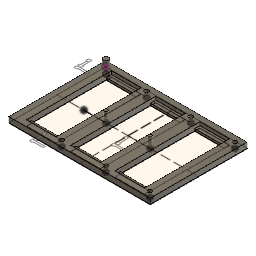
3Slideholder v1 (Autodesk Fusion 360 design; units mm, degrees)
Autodesk Fusion 360 part; units mm, degrees
note: some values were not read from the file. Set by a fixed rule: which sketch regions a step uses.
sketch "Sketch1" plane through (0, 0, 0) normal (0, 1, 0) x (1, 0, 0)
  line L0 (0, 0) -> (127.5, 0)
  line L1 (127.5, 0) -> (127.5, -87.5)
  line L2 (127.5, -87.5) -> (0, -87.5)
  line L3 (0, -87.5) -> (0, 0)
  line L4 (0, -43.75) -> (127.5, -43.75) construction
  line L5 (63.75, 0) -> (63.75, -87.5) construction
  line L6 (63.75, -43.75) -> (77.05, -43.75) construction
  line L7 (63.75, -43.75) -> (63.75, -5.45) construction
  line L8 (63.75, -5.45) -> (77.05, -5.45) construction
  line L9 (77.05, -5.45) -> (50.45, -5.45)
  line L10 (50.45, -5.45) -> (50.45, -82.05)
  line L11 (50.45, -82.05) -> (77.05, -82.05)
  line L12 (77.05, -82.05) -> (77.05, -5.45)
  line L13 (50.45, -43.75) -> (37.25, -43.75)
  line L14 (37.25, -43.75) -> (37.25, -5.45)
  line L15 (37.25, -5.45) -> (10.65, -5.45)
  line L16 (10.65, -5.45) -> (10.65, -82.05)
  line L17 (10.65, -82.05) -> (37.25, -82.05)
  line L18 (37.25, -82.05) -> (37.25, -5.45)
  line L19 (77.05, -43.75) -> (90.25, -43.75)
  line L20 (90.25, -43.75) -> (90.25, -5.45)
  line L21 (90.25, -5.45) -> (116.85, -5.45)
  line L22 (116.85, -5.45) -> (116.85, -82.05)
  line L23 (116.85, -82.05) -> (90.25, -82.05)
  line L24 (90.25, -82.05) -> (90.25, -5.45)
  line L25 (37.25, -43.75) -> (23.95, -43.75)
  line L26 (37.25, -5.45) -> (37.25, -10.2)
  line L27 (37.25, -10.2) -> (10.65, -10.2)
  line L28 (10.65, -10.2) -> (10.65, -5.45)
  line L29 (10.65, -5.45) -> (37.25, -5.45)
  line L30 (37.25, -5.45) -> (37.25, -10.2)
  line L31 (50.45, -5.45) -> (50.45, -10.2)
  line L32 (50.45, -10.2) -> (77.05, -10.2)
  line L33 (77.05, -10.2) -> (77.05, -5.45)
  line L34 (77.05, -5.45) -> (50.45, -5.45)
  line L35 (50.45, -5.45) -> (50.45, -10.2)
  line L36 (90.25, -5.45) -> (90.25, -10.2)
  line L37 (90.25, -10.2) -> (116.85, -10.2)
  line L38 (116.85, -10.2) -> (116.85, -5.45)
  line L39 (116.85, -5.45) -> (90.25, -5.45)
  line L40 (90.25, -5.45) -> (90.25, -10.2)
  line L41 (10.65, -82.05) -> (37.25, -82.05)
  line L42 (37.25, -82.05) -> (37.25, -77.3)
  line L43 (37.25, -77.3) -> (10.65, -77.3)
  line L44 (10.65, -77.3) -> (10.65, -82.05)
  line L45 (50.45, -82.05) -> (77.05, -82.05)
  line L46 (77.05, -82.05) -> (77.05, -77.3)
  line L47 (77.05, -77.3) -> (50.45, -77.3)
  line L48 (50.45, -77.3) -> (50.45, -82.05)
  line L49 (116.85, -82.05) -> (90.25, -82.05)
  line L50 (90.25, -82.05) -> (90.25, -77.3)
  line L51 (90.25, -77.3) -> (116.85, -77.3)
  line L52 (116.85, -77.3) -> (116.85, -82.05)
  line L53 (77.05, -43.75) -> (83.65, -43.75)
  circle A0 centre (83.65, -43.75) radius 1.5
  line L54 (37.25, -43.75) -> (43.85, -43.75)
  circle A1 centre (43.85, -43.75) radius 1.5
  line L55 (10.65, -5.45) -> (5.65, -5.45)
  circle A2 centre (5.65, -5.45) radius 2.5
  line L56 (37.25, -5.45) -> (42.25, -5.45)
  circle A3 centre (42.25, -5.45) radius 1.875
  line L57 (77.05, -5.45) -> (82.05, -5.45)
  circle A4 centre (82.05, -5.45) radius 1.875
  line L58 (116.85, -5.45) -> (121.85, -5.45)
  circle A5 centre (121.85, -5.45) radius 1.875
  line L59 (116.85, -82.05) -> (121.85, -82.05)
  circle A6 centre (121.85, -82.05) radius 1.875
  line L60 (77.05, -82.05) -> (82.05, -82.05)
  circle A7 centre (82.05, -82.05) radius 1.875
  line L61 (37.25, -82.05) -> (42.25, -82.05)
  circle A8 centre (42.25, -82.05) radius 1.875
  dimension "d1" = 127.5
  dimension "d2" = 87.5
  dimension "d3" = 13.3
  dimension "d4" = 38.3
  dimension "d5" = 13.3
  dimension "d6" = 26.6
  dimension "d7" = 76.6
  dimension "d8" = 13.2
  dimension "d9" = 38.3
  dimension "d10" = 26.6
  dimension "d11" = 76.6
  dimension "d12" = 13.2
  dimension "d13" = 38.3
  dimension "d14" = 26.6
  dimension "d15" = 76.6
  dimension "d16" = 13.3
  dimension "d17" = 4.75
  dimension "d18" = 4.75
  dimension "d19" = 4.75
  dimension "d20" = 4.75
  dimension "d21" = 26.6
  dimension "d22" = 4.75
  dimension "d23" = 4.75
  dimension "d42" = 6.6
  dimension "d43" = 3
  dimension "d44" = 6.6
  dimension "d45" = 3
  dimension "d50" = 5
  dimension "d51" = 5
  dimension "d56" = 5
  dimension "d57" = 3.75
  dimension "d58" = 5
  dimension "d59" = 3.75
  dimension "d60" = 5
  dimension "d61" = 3.75
  dimension "d62" = 5
  dimension "d63" = 3.75
  dimension "d64" = 5
  dimension "d65" = 3.75
  dimension "d66" = 5
  dimension "d67" = 3.75
  measures "d4" distance of L0.start
  measures "d7" distance of L0.start
  measures "d9" distance of L0.start
  measures "d11" distance of L0.start
  measures "d13" distance of L0.start
  measures "d15" distance of L0.start
  measures "d43" diameter of A0
  measures "d45" diameter of A1
  measures "d51" diameter of A2
  measures "d57" diameter of A3
  measures "d59" diameter of A4
  measures "d61" diameter of A5
  measures "d63" diameter of A6
  measures "d65" diameter of A7
  measures "d67" diameter of A8
extrude "Extrude12" add sketch "Sketch1" along normal blind 15 contours A2 makes body 1
extrude "Extrude10" add sketch "Sketch1" along normal blind 10 separate body contours L13 L54 A1 | L13 L54 A1 makes body 2
extrude "Extrude1" add sketch "Sketch1" along normal blind 5 separate body contours L0 L1 L2 L3 | L13 L54 A1 | L13 L54 A1 | L19 L53 A0 | L19 L53 A0 | A2 | A3 | A4 | A5 | A6 | A7 | A8 makes body 3
extrude "Extrude2" add sketch "Sketch1" along normal blind 1 contours L20 L21 L22 L24 L36 L37 L38 L39 L40 bodies 3
extrude "Extrude3" add sketch "Sketch1" along normal blind 1 contours L9 L10 L12 L31 L32 L33 L34 L35 bodies 3
extrude "Extrude4" add sketch "Sketch1" along normal blind 2 contours L14 L15 L16 L18 L26 L27 L28 L29 L30 bodies 3
extrude "Extrude5" add 1 faces at (68.1833, 1, 7.0333) along direction (0, 1, 0) blind 1 on bodies 3 bodies 3
extrude "Extrude6" add 1 faces at (107.9833, 1, 8.6167) along direction (0, 1, 0) blind 1 on bodies 3 bodies 3
extrude "Extrude7" add sketch "Sketch1" along normal blind 2 contours L16 L17 L18 L41 L42 L43 L44 bodies 3
extrude "Extrude8" add sketch "Sketch1" along normal blind 2 contours L10 L11 L12 L45 L46 L47 L48 bodies 3
extrude "Extrude9" add sketch "Sketch1" along normal blind 2 contours L22 L23 L24 L49 L50 L51 L52 bodies 3
extrude "Extrude11" add sketch "Sketch1" along normal blind 10 separate body contours L19 L53 A0 | L19 L53 A0 makes body 4
extrude "Extrude13" cut 1 faces at (6.0187, 15, 4.9385) along direction (0, -1, 0) blind 3 on bodies 1 bodies 1
extrude "Extrude14" cut sketch "Sketch1" along normal blind 5 contours A8 bodies 3
extrude "Extrude15" cut sketch "Sketch1" along normal blind 5 contours A7 bodies 3
extrude "Extrude16" cut sketch "Sketch1" along normal blind 5 contours A6 bodies 3
extrude "Extrude17" cut sketch "Sketch1" along normal blind 5 contours A5 bodies 3
extrude "Extrude18" add sketch "Sketch1" along normal blind 1 contours A7 bodies 3
extrude "Extrude19" add sketch "Sketch1" along normal blind 1 contours A8 bodies 3
extrude "Extrude20" add sketch "Sketch1" along normal blind 1 contours A6 bodies 3
extrude "Extrude21" add sketch "Sketch1" along normal blind 1 contours A5 bodies 3
extrude "Extrude22" cut sketch "Sketch1" along normal blind 5 contours A4 bodies 3
extrude "Extrude23" add sketch "Sketch1" along normal blind 1 contours A4 bodies 3
extrude "Extrude24" cut sketch "Sketch1" along normal blind 5 contours A3 bodies 3
extrude "Extrude25" add sketch "Sketch1" along normal blind 1 contours A3 bodies 3
